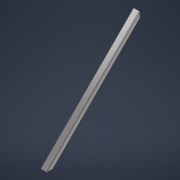
# Autodesk Inventor part: support_truss
Saved by Autodesk Inventor 2021 (Build 250183000, 183)
## iProperties
Created: 2021-05-11
Part Number: support_truss
Material: Steel, Galvanized
Document SubType Name: Modeling
Designer: Watchdog
Density: 7.85 g/cm^3
Appearance: Galvanized
Author: Watchdog
Autodesk Inventor part; units mm, degrees
ref_plane "YZ Plane" through (0, 0, 0) normal (1, 0, 0) x (0, 1, 0)
ref_plane "XZ Plane" through (0, 0, 0) normal (0, 1, 0) x (-1, 0, 0)
sketch "profile" plane through (0, 0, 0) normal (0, 1, 0) x (-1, 0, 0)
  line L0 (12.5, 12.5) -> (-12.5, 12.5)
  line L1 (-12.5, 12.5) -> (-12.5, -12.5)
  line L2 (-12.5, -12.5) -> (12.5, -12.5)
  line L3 (12.5, -12.5) -> (12.5, 12.5)
  line L4 (-10, -10) -> (-10, 10)
  line L5 (-10, 10) -> (10, 10)
  line L6 (10, 10) -> (10, -10)
  line L7 (10, -10) -> (-10, -10)
  point P0 (0, 0)
  dimension "d0" = 12.5
  dimension "d1" = 25
  dimension "d2" = 25
  dimension "d3" = 12.5
  dimension "d6" = 2.5
  constraints: 16 end point, 4 parallel, 2 perpendicular, 1 horizontal, 3 other
  measures "d0" distance from line of point (0, 0) L0
  measures "d1" distance of L2.end L0.start
  measures "d2" distance of L0.start L0.end
  measures "d3" distance from line of point (0, 0) L3
  measures "d6" distance between parallel lines of L1 L4
sketch3d "3D Sketch1"
  line L0 (0, 0, 0) -> (0, 353.5534, -353.5534)
  dimension "d4" = 500
  dimension "d5" = 45
sweep "Sweep1" add profiles "profile" path "3D Sketch1"
fillet "Fillet1" radius 2 4 edges at (-12.5, 176.7767, -189.2767) (-12.5, 176.7767, -164.2767) (12.5, 176.7767, -164.2767) (12.5, 176.7767, -189.2767)
ref_plane "mirrored45" through (-12.5, 353.5534, -341.0534) normal (0, 0, 1) x (1, 0, 0)
split "Split1" plane through (-12.5, 353.5534, -341.0534) removes the side toward (0, 0, -1)
equation "\"d0\" = 0.5 * d1"
equation "\"d1\" = width"
equation "\"d2\" = d1"
equation "\"d3\" = 0.5 * d2"
equation "\"d6\" = t"
equation "\"d4\" = L"
equation "\"d5\" = angleCut"
equation "\"d9\" = filletRadius"
equation "\"t\" = 2.5"
equation "\"filletRadius\" = 2"
equation "\"angleCut\" = 45deg"
equation "\"width\" = 25"
equation "\"a\" = 45"
equation "\"L\" = 500"
body "Solid1"
